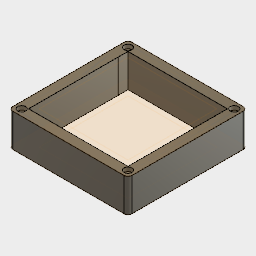
midbody v7 (Autodesk Fusion 360 design; units mm, degrees)
Autodesk Fusion 360 part; units mm, degrees
sketch "Sketch1" plane through (0, 0, 0) normal (0, 1, 0) x (1, 0, 0)
  line L0 (0, 0) -> (89.803, 0)
  line L1 (89.803, 0) -> (89.803, 89.803)
  line L2 (89.803, 89.803) -> (0, 89.803)
  line L3 (0, 89.803) -> (0, 0)
  dimension "d1" = 89.803
  dimension "d2" = 89.803
  measures "d1" distance of L0.start L0.end
  measures "d2" distance of L0.start L2.end
extrude "Extrude1" add sketch "Sketch1" along normal blind 25 makes body 1
sketch "Sketch4" plane through (0, 25, 0) normal (0, 1, 0) x (-1, 0, 0)
  line L0 (0, -89.803) -> (0, 0)
  line L1 (0, 0) -> (-89.803, 0)
  line L2 (-89.803, 0) -> (-89.803, -89.803)
  line L3 (-89.803, -89.803) -> (0, -89.803)
  line L4 (-78.303, -78.303) -> (-11.5, -78.303)
  line L5 (-11.5, -78.303) -> (-11.5, -11.5)
  line L6 (-11.5, -11.5) -> (-78.303, -11.5)
  line L7 (-78.303, -11.5) -> (-78.303, -78.303)
  line L8 (-78.303, -78.303) -> (-11.5, -11.5) construction
  line L9 (-11.5, -78.303) -> (-78.303, -11.5) construction
  point P0 (-44.9015, -44.9015)
  dimension "d10" = 66.803
  dimension "d11" = 66.803
  measures "d10" distance of L5.end L6.end
  measures "d11" distance of L4.end L5.end
extrude "Extrude3" cut sketch "Sketch4" against normal blind 50 contours L4 L5 L6 L7 bodies 1
fillet "Fillet2" radius 3 4 edges at (0, 12.5, 0) (89.803, 12.5, 0) (89.803, 12.5, -89.803) (0, 12.5, -89.803) on bodies 1
sketch "Sketch5" plane through (0, 25, 0) normal (0, 1, 0) x (-1, 0, 0)
  arc A0 (-3, -89.803) -> (0, -86.803) centre (-3, -86.803) ccw
  line L0 (0, -86.803) -> (0, -3)
  arc A1 (0, -3) -> (-3, 0) centre (-3, -3) ccw
  line L1 (-3, 0) -> (-86.803, 0)
  arc A2 (-86.803, 0) -> (-89.803, -3) centre (-86.803, -3) ccw
  line L2 (-89.803, -3) -> (-89.803, -86.803)
  arc A3 (-89.803, -86.803) -> (-86.803, -89.803) centre (-86.803, -86.803) ccw
  line L3 (-86.803, -89.803) -> (-3, -89.803)
  line L4 (-11.5, -78.303) -> (-78.303, -78.303)
  line L5 (-78.303, -78.303) -> (-78.303, -11.5)
  line L6 (-78.303, -11.5) -> (-11.5, -11.5)
  line L7 (-11.5, -11.5) -> (-11.5, -78.303)
copy_body "Body->Comp2" bodies 1 removing the originals makes body 2 in component "midbody2"
sketch "Sketch6" plane through (44.9015, 25, -44.9015) normal (0, 1, 0) x (-1, 0, 0)
  circle A0 centre (-40, 40) radius 3
  circle A1 centre (40, 40) radius 3
  circle A2 centre (-40, -40) radius 3
  circle A3 centre (40, -40) radius 3
  dimension "d15" = 6
  dimension "d16" = 6
  dimension "d17" = 6
  dimension "d18" = 6
  measures "d15" diameter of A0
  measures "d16" diameter of A1
  measures "d17" diameter of A2
  measures "d18" diameter of A3
extrude "Extrude1'" cut sketch "Sketch6" against normal blind 3 bodies 2 in component "midbody2"
sketch "Sketch7" plane through (0, 0, 0) normal (0, -1, 0) x (1, 0, 0)
  line L0 (78.303, -78.303) -> (11.5, -78.303)
  line L1 (11.5, -78.303) -> (11.5, -11.5)
  line L2 (11.5, -11.5) -> (78.303, -11.5)
  line L3 (78.303, -11.5) -> (78.303, -78.303)
  arc A0 (0, -86.803) -> (3, -89.803) centre (3, -86.803) ccw
  line L4 (3, -89.803) -> (86.803, -89.803)
  arc A1 (86.803, -89.803) -> (89.803, -86.803) centre (86.803, -86.803) ccw
  line L5 (89.803, -86.803) -> (89.803, -3)
  arc A2 (89.803, -3) -> (86.803, 0) centre (86.803, -3) ccw
  line L6 (86.803, 0) -> (3, 0)
  arc A3 (3, 0) -> (0, -3) centre (3, -3) ccw
  line L7 (0, -3) -> (0, -86.803)
sketch "Sketch8" plane through (44.9015, 0, -44.9015) normal (0, -1, 0) x (1, 0, 0)
  circle A0 centre (40, 40) radius 3
  circle A1 centre (40, -40) radius 3
  circle A2 centre (40, -40) radius 3
  circle A3 centre (-40, -40) radius 3
  circle A4 centre (-40, 40) radius 3
  point P0 (-37, -40)
  point P1 (-37, 40)
  dimension "d21" = 6
  dimension "d22" = 6
  dimension "d24" = 6
  dimension "d25" = 6
  measures "d21" diameter of A0
  measures "d22" diameter of A1
  measures "d24" diameter of A3
  measures "d25" diameter of A4
extrude "Extrude2" cut sketch "Sketch8" against normal blind 3 bodies 2 in component "midbody2"
sketch "Sketch9" plane through (0, 25, 0) normal (0, 1, 0) x (-1, 0, 0)
  line L0 (-89.803, -3) -> (-89.803, -86.803)
  line L1 (-89.803, -86.803) -> (-89.803, -3)
  line L2 (-86.803, -89.803) -> (-3, -89.803)
  line L3 (0, -86.803) -> (0, -3)
  line L4 (0, -3) -> (0, -86.803)
  line L5 (-3, 0) -> (-86.803, 0)
  line L6 (-86.803, 0) -> (-3, 0)
  line L7 (-75, -7.5) -> (-15, -7.5)
  line L8 (-7.5, -15) -> (-7.5, -75)
  line L9 (-10.5518, -82.303) -> (-78.7446, -82.303)
  line L10 (-82.303, -79.8784) -> (-82.303, -9.9962)
  line L11 (-82.303, -9.9962) -> (-82.303, -7.5)
  line L12 (-82.303, -7.5) -> (-75, -7.5)
  line L13 (-7.5, -15) -> (-7.5, -7.5)
  line L14 (-15, -7.5) -> (-7.5, -7.5)
  line L15 (-7.5, -75) -> (-7.5, -82.303)
  line L16 (-10.5518, -82.303) -> (-7.5, -82.303)
  line L17 (-78.7446, -82.303) -> (-82.303, -82.303)
  line L18 (-82.303, -79.8784) -> (-82.303, -82.303)
extrude "Extrude3'" cut sketch "Sketch9" against normal blind 300 bodies 2 in component "midbody2"
component "midbody2" placed x (1, 0, 0) y (0, 1, 0) z (0, 0, 1) at (0, 0, 0)
